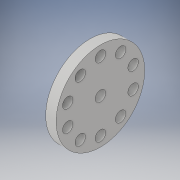
# Autodesk Inventor part: CircularPattern
Saved by Autodesk Inventor 2017 (Build 210142000, 142)
## iProperties
Created: 2020-03-03
Part Number: CircularPattern
Material: Generic
Document SubType Name: Modeling
Designer: 10042265
Density: 1 g/cm^3
Appearance: Default
Author: 10042265
Autodesk Inventor part; units mm, degrees
ref_plane "YZ Plane" through (0, 0, 0) normal (1, 0, 0) x (0, 1, 0)
ref_plane "XZ Plane" through (0, 0, 0) normal (0, 1, 0) x (-1, 0, 0)
ref_plane "XY Plane" through (0, 0, 0) normal (0, 0, 1) x (1, 0, 0)
sketch "Sketch1" plane through (0, 0, 0) normal (0, 0, 1) x (1, 0, 0)
  line L0 (0, 0) -> (0, 15.875)
  line L1 (0, 15.875) -> (12.7, 15.875)
  line L2 (12.7, 15.875) -> (12.7, 53.975)
  line L3 (12.7, 53.975) -> (25.4, 53.975)
  line L4 (25.4, 53.975) -> (25.4, 0)
  line L5 (25.4, 0) -> (0, 0)
  dimension "d0" = 15.875
  dimension "d1" = 12.7
  dimension "d2" = 38.1
  dimension "d3" = 12.7
  constraints: 12 end point, 4 perpendicular, 2 vertical
  measures "d0" distance of L0.start L0.end
  measures "d1" distance of L0.end L1.end
  measures "d2" distance of L1.end L2.end
  measures "d3" distance of L2.end L3.end
revolve "Revolution1" add sketch "Sketch1" angle 360 about axis through (25.4, 0, 0) along (-1, 0, 0)
sketch "Sketch2" plane through (0, 0, 0) normal (-1, 0, 0) x (0, 0, 1)
  point P0 (0, 0)
  point P1 (0, 0)
  constraints: 1 coincident
hole "Hole1" at (0, 0, 0) direction (1, 0, 0) diameter 12.7 end through all
sketch "Sketch3" plane through (12.7, 0, 0) normal (-1, 0, 0) x (0, 0, 1)
  circle A0 centre (0, 0) radius 41.91 construction
  point P0 (0, 83.82)
  point P1 (0, 41.91)
  point P2 (-24.6341, 33.9059)
  point P3 (-39.8588, 12.9509)
  point P4 (-39.8588, -12.9509)
  point P5 (-24.6341, -33.9059)
  point P6 (0, -41.91)
  point P7 (24.6341, -33.9059)
  point P8 (39.8588, -12.9509)
  point P9 (39.8588, 12.9509)
  point P10 (24.6341, 33.9059)
  dimension "d13" = 83.82
  dimension "d16" = 360
  constraints: 1 coincident, 1 vertical alignment, 13 other
hole "Hole2" at (12.7, 83.82, 0) at (12.7, 41.91, 0) at (12.7, 33.9059, -24.6341) at (12.7, 12.9509, -39.8588) at (12.7, -12.9509, -39.8588) at (12.7, -33.9059, -24.6341) at (12.7, -41.91, 0) at (12.7, -33.9059, 24.6341) at (12.7, -12.9509, 39.8588) at (12.7, 12.9509, 39.8588) at (12.7, 33.9059, 24.6341) direction (1, 0, 0) diameter 12.7 end through all
body "Solid1"
